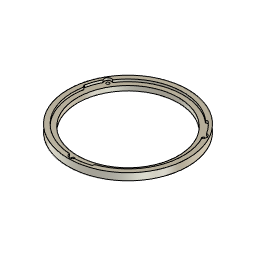
外壳2 v9 (Autodesk Fusion 360 design; units mm, degrees)
Autodesk Fusion 360 part; units mm, degrees
note: some values were not read from the file. Set by a fixed rule: which sketch regions a step uses.
sketch "草图1" plane through (0, 0, 0) normal (0, 0, 1) x (1, 0, 0)
  line L0 (0.9, -43.0906) -> (0.9, -43.1)
  arc A0 (2.5554, -45.5283) -> (2.6381, -48.5283) centre (0, -47.1) ccw
  line L1 (28.4627, -32.3648) -> (28.4702, -32.3737)
  arc A1 (14.7507, -46.3074) -> (13.8402, -43.4489) centre (14.2954, -44.8782) ccw
  line L2 (30.5781, -30.3742) -> (30.6917, -30.5096)
  arc A2 (2.6381, -48.5283) -> (14.7507, -46.3074) centre (0, 0) ccw
  line L3 (42.2601, -8.467) -> (42.2716, -8.469)
  circle A3 centre (0, 0) radius 43.1
  line L4 (11.0158, 41.6685) -> (11.0763, 41.8346)
  arc A4 (-47.4788, 10.3792) -> (-44.548, 9.7385) centre (-46.0134, 10.0589) ccw
  circle A5 centre (40.7898, 23.55) radius 1.25
  line L5 (-11.0158, 41.6685) -> (-11.0763, 41.8346)
  line L6 (-36.8676, 22.3247) -> (-36.8757, 22.3294)
  line L7 (36.8676, 22.3247) -> (36.8757, 22.3294)
  line L8 (-13.7974, 40.8319) -> (-13.8014, 40.8428)
  circle A6 centre (0, 0) radius 47.1 construction
  line L9 (41.5939, -11.2943) -> (41.768, -11.325)
  arc A7 (38.151, 24.9772) -> (30.7078, 33.7104) centre (0, 0) ccw
  arc A8 (-43.3459, 21.9795) -> (-47.4788, 10.3792) centre (0, 0) ccw
  line L10 (-41.5939, -11.2943) -> (-41.768, -11.325)
  line L11 (-28.4627, -32.3648) -> (-28.4702, -32.3737)
  line L12 (-37.7676, 20.7659) -> (-37.7757, 20.7706)
  arc A9 (32.728, 35.9282) -> (30.7078, 33.7104) centre (31.7179, 34.8193) ccw
  arc A10 (-40.7064, 20.5512) -> (-44.548, 9.7385) centre (0, 0) ccw
  circle A11 centre (0, 0) radius 44.72 construction
  arc A12 (40.7077, 26.5489) -> (32.728, 35.9282) centre (0, 0) ccw
  line L13 (-0.9, -43.0906) -> (-0.9, -43.1)
  arc A13 (-40.7064, 20.5512) -> (-43.3459, 21.9795) centre (-40.7898, 23.55) ccw
  arc A14 (38.151, 24.9772) -> (40.7077, 26.5489) centre (40.7898, 23.55) ccw
  circle A15 centre (0, 0) radius 51.1
  line L14 (13.7974, 40.8319) -> (13.8014, 40.8428)
  circle A16 centre (0, -47.1) radius 1.25
  line L15 (-30.5781, -30.3742) -> (-30.6917, -30.5096)
  line L16 (-42.2601, -8.467) -> (-42.2716, -8.469)
  arc A17 (2.5554, -45.5283) -> (13.8402, -43.4489) centre (0, 0) ccw
  circle A18 centre (-40.7898, 23.55) radius 1.25
  line L17 (37.7676, 20.7659) -> (37.7757, 20.7706)
  line L18 (-15.6751, 9.05) -> (-16.3679, 9.45) construction
  line L19 (-37.3257, 21.55) -> (-41.5692, 24) construction
  line L20 (43.1, 0) -> (48, 0) construction
  line L21 (0, -43.1) -> (0, -51.1) construction
  circle A19 centre (0, 0) radius 47.1
  dimension "d17" = 1.8
  dimension "d22" = 6
  dimension "d23" = 3
  dimension "d24" = 2.5
  dimension "d25" = 2.5
  dimension "d26" = 2.5
  dimension "d27" = 86.2
  dimension "d28" = 102.2
  constraint coincident L21.end A15
  constraint coincident A0.centre A6
  constraint coincident A1.centre A6
  constraint tangent A1 A17
  constraint tangent A1 A2
  constraint concentric A0 A16
  constraint concentric A13 A18
  constraint concentric A5 A14
  constraint coincident A3 L14.start
  constraint coincident A3 L5.start
  constraint coincident A3 L8.start
  constraint coincident A3 L4.start
  constraint coincident A3 L12.start
  constraint coincident A3 L6.start
  constraint coincident A3 L19.start
  constraint collinear L18 L19
  constraint coincident A3 L16.start
  constraint coincident A3 L10.start
  constraint coincident A3 L15.start
  constraint coincident A3 L11.start
  constraint coincident A3 L7.start
  constraint coincident A3 L17.start
  constraint coincident A3 L13.start
  constraint coincident A3 L21.start
  constraint coincident A3 L0.start
  constraint coincident A3 L9.start
  constraint coincident A3 L3.start
  constraint coincident A3 L2.start
  constraint coincident A3 L1.start
  constraint concentric A3 A19
  constraint coincident A5.centre A19
  measures "d17" distance of L0 L13
  measures "d22" diameter of A0
  measures "d23" diameter of A1
  measures "d24" diameter of A16
  measures "d25" diameter of A18
  measures "d26" diameter of A5
  measures "d27" diameter of A3
  measures "d28" diameter of A15
extrude "拉伸4" add sketch "草图1" against normal blind 6 contours A0 A1 A16 A17 A19 | A0 A1 A4 A7 A9 A10 A13 A14 A17 A19 | A0 A1 A2 A16 A19 | A4 A10 A13 A18 A19 | A4 A8 A13 A18 A19 | A16 A19 | A16 A19 | A18 A19 | A18 A19 | A5 A9 A12 A14 A19 | A5 A7 A9 A14 A19 | A5 A19 | A5 A19 | A15
extrude "拉伸5" cut sketch "草图1" against normal blind 2 contours A0 A1 A16 A17 A19 | A0 A1 A4 A7 A9 A10 A13 A14 A17 A19 | A0 A1 A2 A16 A19 | A4 A10 A13 A18 A19 | A4 A8 A13 A18 A19 | A16 A19 | A16 A19 | A18 A19 | A18 A19 | A5 A9 A12 A14 A19 | A5 A7 A9 A14 A19 | A5 A19 | A5 A19
extrude "拉伸6" cut sketch "草图1" against normal blind 5 contours A16 A19 | A16 A19 | A18 A19 | A18 A19 | A5 A19 | A5 A19
